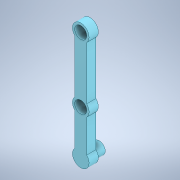
# Autodesk Inventor part: Component27
Saved by Autodesk Inventor 2022 (Build 260153000, 153)
## iProperties
Created: 2022-01-29
Part Number: Component27
Material: Generic
Document SubType Name: Modeling
Designer: Administrator
Density: 1 g/cm^3
Appearance: Default
Title: Component27
Author: Administrator
Autodesk Inventor part; units mm, degrees
ref_plane "YZ Plane" through (0, 0, 0) normal (1, 0, 0) x (0, 1, 0)
ref_plane "XZ Plane" through (0, 0, 0) normal (0, 1, 0) x (-1, 0, 0)
ref_plane "XY Plane" through (0, 0, 0) normal (0, 0, 1) x (1, 0, 0)
sketch "Sketch2" plane through (0, 0, 0) normal (0, 0, 1) x (1, 0, 0)
  circle A0 centre (0, -32.6543) radius 3.25
  circle A1 centre (0, 26.3457) radius 3.25
  circle A2 centre (0, -8.6543) radius 3.25
  line L0 (-3.25, -5.5418) -> (-3.25, 23.2333)
  arc A3 (3.25, 23.2333) -> (-3.25, 23.2333) centre (0, 26.3457) ccw
  arc A4 (3.25, -11.7667) -> (3.25, -5.5418) centre (0, -8.6543) ccw
  arc A5 (-3.25, -29.5418) -> (3.25, -29.5418) centre (0, -32.6543) ccw
  line L1 (-3.25, -29.5418) -> (-3.25, -11.7667)
  arc A6 (-3.25, -5.5418) -> (-3.25, -11.7667) centre (0, -8.6543) ccw
  line L2 (0, 47.7105) -> (0, -62.3205) construction
  line L3 (3.25, -5.5418) -> (3.25, 23.2333)
  line L4 (3.25, -29.5418) -> (3.25, -11.7667)
  point P0 (0, 0)
  dimension "d4" = 6.5
  dimension "d5" = 24
  dimension "d6" = 35
  dimension "d8" = 9
  dimension "d9" = 6.5
  constraints: 10 end point, 8 point on circle, 7 centre point, 5 equal radius, 4 coincident, 4 symmetric about line, 2 point on line, 2 vertical, 1 collinear
  measures "d4" diameter of A2
  measures "d5" distance of A2.centre A0.centre
  measures "d6" distance of A1.centre A2.centre
  measures "d8" diameter of A3
  measures "d9" distance between parallel lines of L1 L4
extrude "Extrusion1" add sketch "Sketch2" along normal blind 5 contours A0 | L0 A3 L3 A4 L4 A5 L1 A6
extrude "Extrusion2" add sketch "Sketch2" against normal blind 5 contours A0
equation "\"d4\" = R"
equation "\"d8\" = R1"
equation "\"d9\" = width"
equation "\"d0\" = thickness"
equation "\"d2\" = thickness"
equation "\"R\" = 6.5"
equation "\"thickness\" = 5"
equation "\"width\" = 6.5"
equation "\"R1\" = 9"
body "Solid1"
